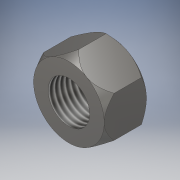
# Autodesk Inventor part: Kingpin_Nut
Saved by Autodesk Inventor 2019 (Build 230136000, 136)
## iProperties
Created: 2020-12-09
Part Number: Kingpin_Nut
Material: Steel, Carbon
Document SubType Name: Modeling
Designer: Anass Hamdi
Density: 7.85 g/cm^3
Appearance: Semi-Polished
Author: Anass Hamdi
Autodesk Inventor part; units mm, degrees
ref_plane "YZ Plane" through (0, 0, 0) normal (1, 0, 0) x (0, 1, 0)
sketch "Sketch1" plane through (0, 0, 0) normal (0, 0, 1) x (1, 0, 0)
  line L0 (0, 8.1984) -> (7.1, 4.0992)
  line L1 (7.1, 4.0992) -> (7.1, -4.0992)
  line L2 (7.1, -4.0992) -> (0, -8.1984)
  line L3 (0, -8.1984) -> (-7.1, -4.0992)
  line L4 (-7.1, -4.0992) -> (-7.1, 4.0992)
  line L5 (-7.1, 4.0992) -> (0, 8.1984)
  point P0 (0, 0)
  point P1 (0, 0)
  dimension "d0" = 14.2
  constraints: 12 end point, 1 coincident, 13 other
  measures "d0" distance between parallel lines of L1 L4
extrude "Extrusion1" add sketch "Sketch1" along normal mid plane 8.5
ref_plane "Work Plane1" through (0, 0, 2.25) normal (0, 0, 1) x (1, 0, 0)
sketch "Sketch2" plane through (0, 0, 4.25) normal (0, 0, 1) x (1, 0, 0)
  arc A0 (-7.1, 0) -> (-3.55, -6.1488) centre (0, 0) ccw
  line L0 (-7.1, 0) -> (-7.1, -4.0992)
  line L1 (-7.1, -4.0992) -> (-3.55, -6.1488)
  constraints: 4 end point, 2 point on circle, 1 centre point, 1 coincident
sketch "Sketch3" plane through (0, 0, 2.25) normal (0, 0, 1) x (1, 0, 0)
  line L0 (-7.1, 4.0992) -> (-7.1, -4.0992) projected
  line L1 (-4.13, -7.0821) -> (-8.2189, -4.6976)
  line L2 (-8.2189, -4.6976) -> (-8.1983, 0.0357)
  arc A0 (-8.1983, 0.0357) -> (-4.13, -7.0821) centre (0, 0) ccw
  constraints: 5 end point, 3 point on circle, 1 centre point, 1 tangent
loft "Loft1" cut profiles "Sketch3", "Sketch2"
pattern_circular "Circular Pattern1" count 6 over 360 about axis through (0, 0, -10) along (0, 0, 1) of "Loft1"
ref_plane "Work Plane2" through (0, 0, -3.25) normal (0, 0, -1) x (-1, 0, 0)
sketch "Sketch4" plane through (0, 0, -4.25) normal (0, 0, -1) x (-1, 0, 0)
  arc A0 (-7.1, 0) -> (-3.55, -6.1488) centre (0, 0) ccw
  line L0 (-7.1, 0) -> (-7.1, -4.0992)
  line L1 (-7.1, -4.0992) -> (-3.55, -6.1488)
  constraints: 4 end point, 2 point on circle, 1 centre point, 1 coincident
sketch "Sketch5" plane through (0, 0, -3.25) normal (0, 0, -1) x (-1, 0, 0)
  line L0 (-4.13, -7.0821) -> (-8.2189, -4.6976)
  line L1 (-8.2189, -4.6976) -> (-8.1983, 0.0357)
  arc A0 (-8.1983, 0.0357) -> (-4.13, -7.0821) centre (0, 0) ccw
  constraints: 4 end point, 2 point on circle, 1 centre point, 1 tangent
loft "Loft2" cut profiles "Sketch4", "Sketch5"
pattern_circular "Circular Pattern2" count 6 over 360 about axis through (0, 0, -10) along (0, 0, 1) of "Loft2"
sketch "Sketch6" plane through (0, 0, 4.25) normal (0, 0, 1) x (1, 0, 0)
  point P0 (0, 0)
  point P1 (0, 0)
  constraints: 1 coincident
hole "Hole1" at (0, 0, 4.25) direction (0, 0, -1) diameter 8.382 depth 8.5 thread size "3/8-24 UNF" class "2B" standard "ANSI Unified Screw Threads"
body "Solid1"
